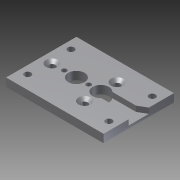
# Autodesk Inventor part: 13_1087_012
Saved by Autodesk Inventor 2014 SP1 (Build 180222100, 222)
## iProperties
Created: 2013-08-08
Part Number: 13_1087_012
Material: Allgemein
Document SubType Name: Modeling
Designer: vogel
Density: 1 g/cm^3
Appearance: Vorgabe
Author: vogel
Autodesk Inventor part; units mm, degrees
ref_plane "YZ Plane" through (0, 0, 0) normal (1, 0, 0) x (0, 1, 0)
ref_plane "XZ Plane" through (0, 0, 0) normal (0, 1, 0) x (-1, 0, 0)
ref_plane "XY Plane" through (0, 0, 0) normal (0, 0, 1) x (1, 0, 0)
sketch "Skizze1" plane through (0, 0, 0) normal (0, 0, 1) x (1, 0, 0)
  line L0 (-7.2, 0) -> (43.2, 0) projected
  line L1 (0, -4.6) -> (0, 27.6) projected
  line L2 (0, 23) -> (36, 23)
  line L3 (36, 23) -> (36, 0)
  line L4 (36, 0) -> (0, 0)
  line L5 (0, 0) -> (0, 23)
  point P0 (0, 0)
  dimension "d0" = 36
  dimension "d1" = 23
  constraints: 8 end point, 2 collinear, 2 parallel, 1 horizontal, 1 perpendicular
  measures "d0" distance of L2.start L2.end
  measures "d1" distance of L2.end L3.end
extrude "Extrusion1" add sketch "Skizze1" along normal blind 3
hole "Bohrung1" at (13, 13, 0) direction (0, 0, 1) diameter 6 end through all
sketch "Skizze3" plane through (0, 0, 3) normal (0, 0, 1) x (1, 0, 0)
  line L0 (19, 18) -> (7, 18) projected
  line L1 (7, 18) -> (7, 8) projected
  line L2 (19, 8) -> (19, 18) projected
  line L3 (7, 8) -> (19, 8) projected
  circle A0 centre (17, 16) radius 1.25 projected
  circle A1 centre (9, 10) radius 1.25 projected
  circle A2 centre (17.5, 13) radius 0.6105 projected
  circle A3 centre (8.5, 13) radius 0.6105 projected
  point P0 (8.5, 13)
  point P1 (17.5, 13)
hole "Bohrung2" at (8.5, 13, 3) at (17.5, 13, 3) direction (0, 0, -1) diameter 1.8 end through all
sketch "Skizze5" plane through (0, 0, 0) normal (0, 0, -1) x (-1, 0, 0)
  circle A0 centre (-17, 16) radius 1.25 projected
  circle A1 centre (-9, 10) radius 1.25 projected
  point P0 (-17, 16)
  point P1 (-9, 10)
hole "Bohrung3" at (17, 16, 0) at (9, 10, 0) direction (0, 0, 1) diameter 3.5 depth 1 tip angle 118
sketch "Skizze6" plane through (0, 23, 0) normal (0, 1, 0) x (1, 0, 0)
  line L0 (0, 0) -> (36, 0) projected
  line L1 (0, 0) -> (0, -3) projected
  line L2 (36, -3) -> (0, -3) projected
  line L3 (36, 0) -> (36, -3) projected
extrude "Extrusion2" add sketch "Skizze6" along normal blind 3
sketch "Skizze7" plane through (0, 0, 0) normal (0, 0, -1) x (-1, 0, 0)
  line L0 (-36, 26) -> (-36, 0) projected
  line L1 (-36, 0) -> (0, 0) projected
  line L2 (0, 0) -> (0, 26) projected
  line L3 (-36, 26) -> (0, 26) projected
  line L4 (-36, 25.9998) -> (0, 25.9998) projected
  line L5 (-6, 23) -> (-6, 3) projected
  line L6 (-26, 3) -> (-26, 23) projected
  line L7 (-36, 23) -> (0, 23) projected
  line L8 (0, 0) -> (-36, 0) projected
  line L9 (-6, 3) -> (-26, 3) projected
  line L10 (-6.5, 9) -> (-6.5, 17) projected
  arc A0 (-6.5, 17) -> (-8, 18.5) centre (-8, 17) ccw projected
  line L11 (-8, 18.5) -> (-10.0314, 18.5) projected
  line L12 (-15.9686, 18.5) -> (-18, 18.5) projected
  arc A1 (-18, 18.5) -> (-19.5, 17) centre (-18, 17) ccw projected
  line L13 (-19, 8) -> (-19, 18) projected
  line L14 (-16.2253, 8) -> (-19, 8) projected
  line L15 (-19.5, 17) -> (-19.5, 16) projected
  arc A2 (-19.5, 16) -> (-18, 7.5) centre (-18, 9) ccw projected
  arc A3 (-10.0314, 7.5) -> (-10.0314, 18.5) centre (-13, 13) ccw projected
  line L16 (-18, 7.5) -> (-15.9686, 7.5) projected
  line L17 (-10.0314, 7.5) -> (-8, 7.5) projected
  arc A4 (-8, 7.5) -> (-6.5, 9) centre (-8, 9) ccw projected
  line L18 (-6.5, 9) -> (-6.5, 17) projected
  line L19 (-3, 0) -> (-3, 25.9998)
  line L20 (-33, 25.9998) -> (-33, 0)
  line L21 (-33, 21) -> (-3, 21)
  line L22 (-3, 21) -> (-3, 5)
  line L23 (-3, 5) -> (-33, 5)
  line L24 (-33, 5) -> (-33, 21)
  line L25 (-36, 13) -> (0, 13)
  point P0 (-6, 23)
  dimension "d29" = 6
  dimension "d30" = 3
  dimension "d31" = 3
  dimension "d32" = 16
  constraints: 14 end point, 6 point on line, 3 perpendicular, 2 coincident, 2 midpoint, 2 parallel, 1 horizontal, 6 other
  measures "d30" distance between parallel lines of L2 L19
  measures "d31" distance between parallel lines of L0 L20
  measures "d32" distance between parallel lines of L23 L21
hole "Bohrung4" at (3, 21, 0) at (3, 5, 0) at (33, 21, 0) at (33, 5, 0) direction (0, 0, 1) diameter 2.4 end through all countersink diameter 4.5 countersink angle 90
sketch "Skizze9" plane through (0, 0, 3) normal (0, 0, 1) x (1, 0, 0)
  line L0 (0, 0) -> (0, 26) projected
  line L1 (36, 0) -> (36, 26) projected
  line L2 (3, 8) -> (2, 8) projected
  line L3 (2, 8) -> (2, 18) projected
  line L4 (2, 18) -> (3, 18) projected
  arc A0 (3, 18) -> (6, 21) centre (3, 21) ccw projected
  line L5 (6, 21) -> (6, 23) projected
  line L6 (6, 3) -> (6, 5) projected
  arc A1 (6, 5) -> (3, 8) centre (3, 5) ccw projected
  line L7 (0, 13) -> (36, 13)
  line L8 (22, 20.2065) -> (22, 3.5507)
  line L9 (6, 23) -> (30, 23) projected
  line L10 (30, 3) -> (30, 5) projected
  line L11 (6, 3) -> (30, 3) projected
  arc A2 (30, 21) -> (33, 18) centre (33, 21) ccw projected
  line L12 (34, 18) -> (33, 18) projected
  line L13 (34, 8) -> (34, 18) projected
  line L14 (33, 8) -> (34, 8) projected
  arc A3 (33, 8) -> (30, 5) centre (33, 5) ccw projected
  line L15 (30, 21) -> (30, 23) projected
  point P0 (22, 19)
  point P1 (22, 7)
  point P2 (4, 13)
  dimension "d41" = 22
  dimension "d42" = 14
  dimension "d43" = 12
  dimension "d44" = 4
  constraints: 4 end point, 3 point on line, 2 midpoint, 1 perpendicular, 1 symmetric about line
  measures "d41" distance between parallel lines of L8 L0
  measures "d42" distance between parallel lines of L1 L8
  measures "d43" distance of point (22, 7) point (22, 19)
  measures "d44" distance from line of point (4, 13) L0
hole "Bohrung5" at (22, 19, 3) at (22, 7, 3) at (4, 13, 3) direction (0, 0, -1) diameter 2.4 end through all countersink diameter 4.5 countersink angle 90
sketch "Skizze10" plane through (0, 0, 3) normal (0, 0, 1) x (1, 0, 0)
  circle A0 centre (22, 19) radius 2.25 projected
  line L0 (36, 0) -> (36, 26) projected
  line L1 (0, 26) -> (36, 26) projected
  line L2 (36, 13) -> (19.5709, 13)
  line L3 (36, 11) -> (22, 11)
  line L4 (36, 15) -> (22, 15)
  line L5 (22, 15) -> (22, 11)
  line L6 (22, 19) -> (22, 15.7462)
  dimension "d52" = 4
  constraints: 10 end point, 3 parallel, 2 collinear, 2 point on line, 1 midpoint, 1 vertical, 1 other
  measures "d52" distance between parallel lines of L3 L4
extrude "Extrusion3" cut sketch "Skizze10" against normal blind 2 contours L3 L5 L2 L0 | L2 L5 L4 L0
sketch "Skizze11" plane through (0, 0, 3) normal (0, 0, 1) x (1, 0, 0)
  line L0 (22, 11) -> (22, 15) projected
  point P0 (22, 13)
  constraints: 1 midpoint
hole "Bohrung6" at (22, 13, 3) direction (0, 0, -1) diameter 6 end through all
chamfer "Fase1" distance 3 angle 30 1 edges at (36, 11, 2) measured on face at (28.1574, 11, 2.3333)
chamfer "Fase2" distance 3 angle 30 1 edges at (36, 15, 2) measured on face at (32.0787, 15, 2.3333)
